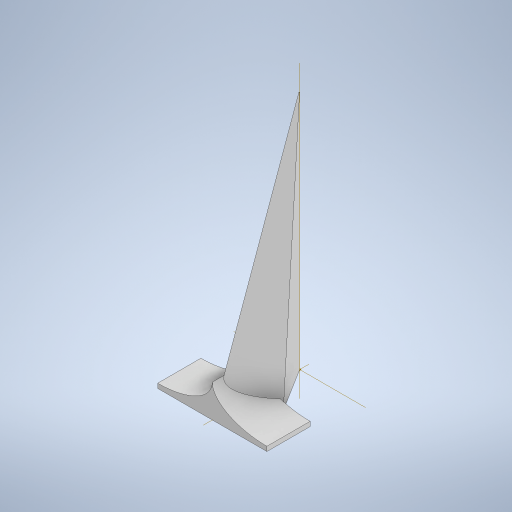
# Autodesk Inventor part: Plough
Saved by Autodesk Inventor 2023.2 (Build 272271030, 271C)
## iProperties
Created: 2023-02-16
Part Number: Plough
Material: Generisch
Document SubType Name: Modeling
Designer: mehan
Density: 1 g/cm^3
Appearance: Vorgabe
Author: mehan
Autodesk Inventor part; units mm, degrees
ref_plane "YZ Plane" through (0, 0, 0) normal (1, 0, 0) x (0, 1, 0)
ref_plane "XZ Plane" through (0, 0, 0) normal (0, 1, 0) x (-1, 0, 0)
ref_plane "XY Plane" through (0, 0, 0) normal (0, 0, 1) x (1, 0, 0)
sketch "Skizze1" plane through (0, 0, 0) normal (0, 1, 0) x (-1, 0, 0)
  line L0 (0, 40) -> (-25, 0)
  line L1 (0, 40) -> (25, 0)
  line L2 (0, -40) -> (-25, 0)
  line L3 (0, -40) -> (25, 0)
  point P0 (0, 0)
  dimension "d0" = 25
  dimension "d1" = 40
  dimension "d6" = 40
  constraints: 8 end point
  measures "d0" distance of point (0, 0) L0.end
  measures "d1" distance of point (0, 0) L0.start
  measures "d6" distance of point (0, 0) L2.start
extrude "Extrusion3" add sketch "Skizze1" along normal blind 110 draft -10.8
sketch "Skizze3" plane through (0, 0, 0) normal (0, -1, 0) x (1, 0, 0)
  line L0 (25, 0) -> (0.2551, 0) projected
  line L1 (-25.0005, 0) -> (25, 0)
  line L2 (0, 40) -> (25, 0) projected
  line L3 (25, 0) -> (0, -40) projected
  line L4 (25, 0) -> (0, -40)
  line L5 (0, -40) -> (-25.0005, 0)
  point P0 (0, 0)
  constraints: 6 end point, 2 collinear
extrude "Extrusion4" cut sketch "Skizze3" against normal blind 110
sketch "Skizze4" plane through (0, 0, 0) normal (0, -1, 0) x (1, 0, 0)
  line L0 (-25, 0) -> (0, 40) projected
  line L1 (-12.5, 20) -> (0, 0)
  line L2 (-25, 0) -> (25, 0) projected
  line L3 (0, 0) -> (-25, 0)
  line L4 (-25, 0) -> (-12.5, 20)
  constraints: 6 end point, 1 collinear, 1 midpoint
extrude "Extrusion5" cut sketch "Skizze4" against normal blind 110
sketch "Skizze5" plane through (0, 0, 0) normal (0, -1, 0) x (1, 0, 0)
  line L0 (0, 40) -> (25, 0) projected
  line L1 (12.5, 20) -> (0, 0)
  line L2 (25, 0) -> (0.2551, 0) projected
  line L3 (0, 0) -> (25, 0)
  line L4 (25, 0) -> (12.5, 20)
  constraints: 6 end point, 1 collinear, 1 midpoint
extrude "Extrusion6" cut sketch "Skizze5" against normal blind 110
sketch "Skizze6" plane through (0, 0, 0) normal (0, 1, 0) x (-1, 0, 0)
  line L0 (0, 40) -> (0, 0.4082) projected
  line L1 (0, 40) -> (-25, 40)
  line L2 (-25, 40) -> (-25, 20.2041)
  line L3 (-25, 20.2041) -> (25, 20.2041)
  line L4 (25, 20.2041) -> (25, 40)
  line L5 (25, 40) -> (0, 40)
  point P0 (0, 0)
  dimension "d15" = 25
  dimension "d16" = 50
  constraints: 10 end point, 4 perpendicular, 1 horizontal, 1 point on line
  measures "d15" distance of L0.start L1.end
  measures "d16" distance of L2.end L3.end
extrude "Extrusion7" add sketch "Skizze6" along normal blind 15
sketch "Skizze7" plane through (-25, 0, 40) normal (0, 0, 1) x (1, 0, 0)
  line L0 (25, 0) -> (25, 110) projected
  line L1 (0, 0) -> (0, 15) projected
  ellipse E0 centre (0, 15) end of major axis (25, 15) minor radius 12.9109 (0, 2.0891) -> (25, 15) ccw
  ellipse E1 centre (50, 15) end of major axis (25, 15) minor radius 12.9109 (25, 15) -> (50, 2.0891) ccw
  line L2 (50, 2.0891) -> (50, 15)
  line L3 (25, 15) -> (33.9981, 15) projected
  line L4 (50, 15) -> (25, 15)
  line L5 (0, 15) -> (50, 15) projected
  line L6 (25, 15) -> (0, 15)
  line L7 (0, 15) -> (0, 2.0891)
  constraints: 8 end point, 2 perpendicular, 2 point on line, 2 symmetric about line, 2 vertical, 1 coincident, 1 collinear, 8 other
extrude "Extrusion8" cut sketch "Skizze7" along normal up to surface contours L3 L4 L2 E1 surface through (25, 0, 0) normal (0.8329779, 0.1873813, 0.5206112)
extrude "Extrusion9" cut sketch "Skizze7" against normal up to surface contours L1 L5 E0 surface through (0, 0, 40) normal (-0.8329779, 0.1873813, 0.5206112)
